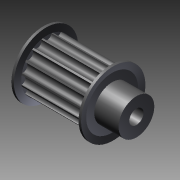
# Autodesk Inventor part: zrr_htd_3m15_4_17031600
Saved by Autodesk Inventor 2011 SP1 (Build 150282100, 282)
## iProperties
Created: 2018-07-07
Part Number: zrr_htd_3m15_4_17031600
Catalog Web Link: www.cadenas.de
Description: zrr_htd_3m15-HTD Pulleys Profile 3M, Timing Belt Width 15mm
Vendor: MAEDLER
Document SubType Name: Modeling
Designer: psAdmin
Manufacturer: MAEDLER
Mass: 8.5 g
Surface Area: 24.7998 cm^2
Volume: 2.91131 cm^3
Density: 1 g/cm^3
Category: PARTsolutions
Company: MAEDLER
Title: zrr_htd_3m15_4_17031600
Author: Cadenas PARTsolutions
Comments: HTD Pulleys Profile 3M, Timing Belt Width 15mm
PSOL_IDENT_0: {$CADENAS_DATA\23d-libs\maedler\antriebselemente\zahnriemenraeder_zahnriemen\zahnriemenraeder\htd-pr
PSOL_IDENT_1: ofil\zrr_htd_3m15.prj},197 {VTYP=3D},{NB=zrr_htd_3m15_4_17031600},{LINA=zrr_htd_3m15_4_17031600},{NN=
PSOL_IDENT_2: zrr_htd_3m15},{DATE=16.06.2017 10:47:49},{GEOMDATE=09.06.2016 09:07:07},{VERSION=},{LINEID=250},{LIN
PSOL_IDENT_3: ESUBID=-1},{WBVAR=BX}  {NB=zrr_htd_3m15_4_17031600},{LINA=zrr_htd_3m15_4_17031600},{KT=DUMMY},{ARTNR=
PSOL_IDENT_4: 17031600},{PDF=PDF Katalogseite},{AUSF=16-3M-15-1F},{MAT=Aluminium},{ZTL=3.000},{ZRB=15.000},{Z=16.0
PSOL_IDENT_5: 00},{AUS=1F},{ZS=14.520},{BS=18.000},{DO=15.280},{ND=10.000},{B=19.500},{L=26.000},{I=0.000},{VB=4.0
PSOL_IDENT_6: 00},{FB=5.500},{BX=4},{GEW=8.500},{ZT=1.200},{ZB=1.800},{T=1.000},{BB=1.000}
NN: zrr_htd_3m15
NT: HTD-Zahnriemenräder Profil 3M, Zahnriemenbreite 15mm
NB: zrr_htd_3m15_4_17031600
NBSYN: zrr_htd_3m15_$BX._$ARTNR.
LINA: zrr_htd_3m15_4_17031600
ARTNR: 17031600
PDF: PDF Katalogseite
AUSF: 16-3M-15-1F
MAT: Aluminium
ZTL: 3.000
ZRB: 15.000
Z: 16.000
AUS: 1F
ZS: 14.520
BS: 18.000
DO: 15.280
ND: 10.000
B: 19.500
L: 26.000
I: 0.000
VB: 4.000
FB: 5.500
BX: 4
GEW: 8.500
ZT: 1.200
ZB: 1.800
T: 1.000
BB: 1.000
SUPPLIER: MAEDLER
ARTICLENO: zrr_htd_3m15_4_17031600
BOMINFO: zrr_htd_3m15_4_17031600
CREATOR: CADENAS GmbH
Autodesk Inventor part; units mm, degrees
ref_plane "YZ Plane" through (0, 0, 0) normal (1, 0, 0) x (0, 1, 0)
ref_plane "XZ Plane" through (0, 0, 0) normal (0, 1, 0) x (-1, 0, 0)
ref_plane "XY Plane" through (0, 0, 0) normal (0, 0, 1) x (1, 0, 0)
sketch "Sketch_3" plane through (0, 0, 0) normal (0, 0, 1) x (1, 0, 0)
  line L0 (500, 0) -> (-500, 0)
  line L1 (0, 0) -> (0, 9)
  line L2 (0, 9) -> (0.6932, 9)
  line L3 (0.6932, 9) -> (1, 7.26)
  line L4 (1, 7.26) -> (18.5, 7.26)
  line L5 (18.5, 7.26) -> (18.8068, 9)
  line L6 (18.8068, 9) -> (19.5, 9)
  line L7 (19.5, 9) -> (19.1932, 7.26)
  line L8 (19.1932, 7.26) -> (19.1932, 5)
  line L9 (19.1932, 5) -> (26, 5)
  line L10 (26, 5) -> (26, 0)
  line L11 (26, 0) -> (0, 0)
  constraints: 24 end point
revolve "Revolution1" add sketch "Sketch_3" angle 360 about axis through (500, 0, 0) along (1, 0, 0)
sketch "Sketch_4" plane through (1, 0, 0) normal (1, 0, 0) x (0, 0, -1)
  circle A0 centre (0, 0) radius 260
  arc A1 (-7.1608, -1.1959) -> (-7.1205, -1.4164) centre (0, 0) ccw
  arc A2 (-7.1205, -1.4164) -> (-7.0734, -1.6355) centre (0, 0) ccw
  arc A3 (-6.1581, -3.8452) -> (-7.0734, -1.6355) centre (-6.7074, -2.7783) ccw
  arc A4 (-6.1581, -3.8452) -> (-6.0365, -4.0334) centre (0, 0) ccw
  arc A5 (-6.0365, -4.0334) -> (-5.9091, -4.2178) centre (0, 0) ccw
  arc A6 (-4.2178, -5.9091) -> (-5.9091, -4.2178) centre (-5.1336, -5.1336) ccw
  arc A7 (-4.2178, -5.9091) -> (-4.0334, -6.0365) centre (0, 0) ccw
  arc A8 (-4.0334, -6.0365) -> (-3.8452, -6.1581) centre (0, 0) ccw
  arc A9 (-1.6355, -7.0734) -> (-3.8452, -6.1581) centre (-2.7783, -6.7074) ccw
  arc A10 (-1.6355, -7.0734) -> (-1.4164, -7.1205) centre (0, 0) ccw
  arc A11 (-1.4164, -7.1205) -> (-1.1959, -7.1608) centre (0, 0) ccw
  arc A12 (1.1959, -7.1608) -> (-1.1959, -7.1608) centre (0, -7.26) ccw
  arc A13 (1.1959, -7.1608) -> (1.4164, -7.1205) centre (0, 0) ccw
  arc A14 (1.4164, -7.1205) -> (1.6355, -7.0734) centre (0, 0) ccw
  arc A15 (3.8452, -6.1581) -> (1.6355, -7.0734) centre (2.7783, -6.7074) ccw
  arc A16 (3.8452, -6.1581) -> (4.0334, -6.0365) centre (0, 0) ccw
  arc A17 (4.0334, -6.0365) -> (4.2178, -5.9091) centre (0, 0) ccw
  arc A18 (5.9091, -4.2178) -> (4.2178, -5.9091) centre (5.1336, -5.1336) ccw
  arc A19 (5.9091, -4.2178) -> (6.0365, -4.0334) centre (0, 0) ccw
  arc A20 (6.0365, -4.0334) -> (6.1581, -3.8452) centre (0, 0) ccw
  arc A21 (7.0734, -1.6355) -> (6.1581, -3.8452) centre (6.7074, -2.7783) ccw
  arc A22 (7.0734, -1.6355) -> (7.1205, -1.4164) centre (0, 0) ccw
  arc A23 (7.1205, -1.4164) -> (7.1608, -1.1959) centre (0, 0) ccw
  arc A24 (7.1608, 1.1959) -> (7.1608, -1.1959) centre (7.26, 0) ccw
  arc A25 (7.1608, 1.1959) -> (7.1205, 1.4164) centre (0, 0) ccw
  arc A26 (7.1205, 1.4164) -> (7.0734, 1.6355) centre (0, 0) ccw
  arc A27 (6.1581, 3.8452) -> (7.0734, 1.6355) centre (6.7074, 2.7783) ccw
  arc A28 (6.1581, 3.8452) -> (6.0365, 4.0334) centre (0, 0) ccw
  arc A29 (6.0365, 4.0334) -> (5.9091, 4.2178) centre (0, 0) ccw
  arc A30 (4.2178, 5.9091) -> (5.9091, 4.2178) centre (5.1336, 5.1336) ccw
  arc A31 (4.2178, 5.9091) -> (4.0334, 6.0365) centre (0, 0) ccw
  arc A32 (4.0334, 6.0365) -> (3.8452, 6.1581) centre (0, 0) ccw
  arc A33 (1.6355, 7.0734) -> (3.8452, 6.1581) centre (2.7783, 6.7074) ccw
  arc A34 (1.6355, 7.0734) -> (1.4164, 7.1205) centre (0, 0) ccw
  arc A35 (1.4164, 7.1205) -> (1.1959, 7.1608) centre (0, 0) ccw
  arc A36 (-1.1959, 7.1608) -> (1.1959, 7.1608) centre (0, 7.26) ccw
  arc A37 (-1.1959, 7.1608) -> (-1.4164, 7.1205) centre (0, 0) ccw
  arc A38 (-1.4164, 7.1205) -> (-1.6355, 7.0734) centre (0, 0) ccw
  arc A39 (-3.8452, 6.1581) -> (-1.6355, 7.0734) centre (-2.7783, 6.7074) ccw
  arc A40 (-3.8452, 6.1581) -> (-4.0334, 6.0365) centre (0, 0) ccw
  arc A41 (-4.0334, 6.0365) -> (-4.2178, 5.9091) centre (0, 0) ccw
  arc A42 (-5.9091, 4.2178) -> (-4.2178, 5.9091) centre (-5.1336, 5.1336) ccw
  arc A43 (-5.9091, 4.2178) -> (-6.0365, 4.0334) centre (0, 0) ccw
  arc A44 (-6.0365, 4.0334) -> (-6.1581, 3.8452) centre (0, 0) ccw
  arc A45 (-7.0734, 1.6355) -> (-6.1581, 3.8452) centre (-6.7074, 2.7783) ccw
  arc A46 (-7.0734, 1.6355) -> (-7.1205, 1.4164) centre (0, 0) ccw
  arc A47 (-7.1205, 1.4164) -> (-7.1608, 1.1959) centre (0, 0) ccw
  arc A48 (-7.1608, -1.1959) -> (-7.1608, 1.1959) centre (-7.26, 0) ccw
  constraints: 96 point on circle, 49 centre point
extrude "Extrusion1" cut sketch "Sketch_4" along normal blind 17.5
sketch "Sketch_9_ALT_Drilling_1" plane through (0, 0, 0) normal (1, 0, 0) x (0, 1, 0)
  circle A0 centre (0, 0) radius 2
  constraints: 1 centre point
extrude "Extrusion2" cut sketch "Sketch_9_ALT_Drilling_1" along normal blind 26
body "Solid1"
